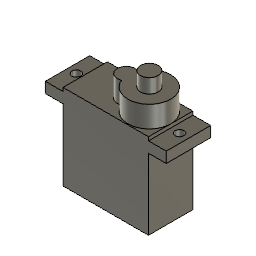
SG90 (Autodesk Fusion 360 design; units mm, degrees)
part number: 2026-08-23-17-35-19-332
Autodesk Fusion 360 part; units mm, degrees
note: some values were not read from the file. Set by a fixed rule: which sketch regions a step uses.
sketch "Sketch1" plane through (0, 0, 0) normal (0, 0, 1) x (1, 0, 0)
  line L0 (12, 6.25) -> (-12, 6.25)
  line L1 (-12, 6.25) -> (-12, -6.25)
  line L2 (-12, -6.25) -> (12, -6.25)
  line L3 (12, -6.25) -> (12, 6.25)
  line L4 (12, 6.25) -> (-12, -6.25) construction
  line L5 (-12, 6.25) -> (12, -6.25) construction
  line L6 (12, 6.25) -> (17, 6.25)
  line L7 (17, 6.25) -> (17, -6.25)
  line L8 (12, -6.25) -> (17, -6.25)
  line L9 (-12, 6.25) -> (-17, 6.25)
  line L10 (-17, 6.25) -> (-17, -6.25)
  line L11 (-17, -6.25) -> (-12, -6.25)
  dimension "d1" = 24
  dimension "d2" = 12.5
  dimension "d3" = 5
  dimension "d4" = 5
  constraint horizontal L0
  constraint perpendicular L0 L1
  constraint parallel L0 L2
  constraint parallel L1 L3
  constraint coincident L4 origin
  constraint coincident L5 origin
  constraint perpendicular L3 L6
  constraint perpendicular L2 L7
  constraint perpendicular L7 L8
  constraint perpendicular L1 L9
  constraint perpendicular L0 L10
  constraint perpendicular L1 L11
  measures "d1" distance of L1.end L2.end
  measures "d2" distance of L0.end L1.end
  measures "d3" distance of L0.start L6.end
  measures "d4" distance of L0.end L9.end
extrude "Extrude1" add sketch "Sketch1" along normal blind 24 contours L0 L1 L2 L3
sketch "Sketch2" plane through (0, -6.25, 0) normal (0, -1, 0) x (1, 0, 0)
  line L0 (-12, 0) -> (12, 0)
  line L1 (12, 0) -> (12, 24)
  line L2 (12, 24) -> (-12, 24)
  line L3 (-12, 24) -> (-12, 0)
  line L4 (12, 24) -> (12, 23)
  line L5 (12, 23) -> (17, 23)
  line L6 (17, 23) -> (17, 20)
  line L7 (17, 20) -> (12, 20)
  line L8 (-12, 24) -> (-12, 23)
  line L9 (-12, 23) -> (-17, 23)
  line L10 (-17, 23) -> (-17, 20)
  line L11 (-17, 20) -> (-12, 20)
  dimension "d7" = 1
  dimension "d8" = 5
  dimension "d9" = 3
  dimension "d10" = 1
  dimension "d11" = 5
  dimension "d12" = 3
  constraint coincident L1.end L2.start
  constraint perpendicular L2 L4
  constraint perpendicular L1 L5
  constraint perpendicular L5 L6
  constraint coincident L1 L7.end
  constraint perpendicular L1 L7
  constraint coincident L2.end L3.start
  constraint perpendicular L2 L8
  constraint perpendicular L3 L9
  constraint perpendicular L9 L10
  constraint coincident L3 L11.end
  constraint perpendicular L3 L11
  measures "d7" distance of L1.end L4.end
  measures "d8" distance of L4.end L5.end
  measures "d9" distance of L5.end L6.end
  measures "d10" distance of L2.end L8.end
  measures "d11" distance of L8.end L9.end
  measures "d12" distance of L9.end L10.end
extrude "Extrude2" add sketch "Sketch2" against normal up to surface (12.5 mm away) contours L3 L9 L10 L11 | L1 L5 L6 L7
sketch "Sketch3" plane through (0, 0, 24) normal (0, 0, 1) x (-1, 0, 0)
  line L0 (-12, 6.25) -> (-12, -6.25)
  line L1 (-12, -6.25) -> (12, -6.25)
  line L2 (12, -6.25) -> (12, 6.25)
  line L3 (12, 6.25) -> (-12, 6.25)
  circle A0 centre (-6, 0) radius 6
  circle A1 centre (0.5, 0) radius 2.5
  dimension "d15" = 12
  dimension "d16" = 5
  dimension "d17" = 6.5
  constraint tangent L0 A0
  measures "d15" diameter of A0
  measures "d16" diameter of A1
  measures "d17" distance of A0.centre A1.centre
extrude "Extrude3" add sketch "Sketch3" along normal blind 6 contours A0 A1 | A0 A1 | A0 A1
sketch "Sketch4" plane through (0, 0, 30) normal (0, 0, 1) x (-1, 0, 0)
  arc A0 (-0.4615, -2.3077) -> (-0.4615, 2.3077) centre (0.5, 0) ccw
  arc A1 (-0.4615, 2.3077) -> (-0.4615, -2.3077) centre (-6, 0) ccw
  circle A2 centre (-6, 0) radius 2.5
  dimension "d20" = 5
  constraint concentric A1 A2
  measures "d20" diameter of A2
extrude "Extrude4" add sketch "Sketch4" along normal blind 4 contours A2
sketch "Sketch5" plane through (0, 0, 23) normal (0, 0, 1) x (-1, 0, 0)
  line L0 (-17, -6.25) -> (-12, -6.25)
  line L1 (-12, -6.25) -> (-12, 6.25)
  line L2 (-12, 6.25) -> (-17, 6.25)
  line L3 (-17, 6.25) -> (-17, -6.25)
  circle A0 centre (-14.5, 0) radius 1.25
  dimension "d23" = 2.5
  dimension "d24" = 2.5
  measures "d23" diameter of A0
  measures "d24" distance of L3 A0.centre
sketch "Sketch6" plane through (0, 0, 23) normal (0, 0, 1) x (-1, 0, 0)
  line L0 (12, -6.25) -> (17, -6.25)
  line L1 (17, -6.25) -> (17, 6.25)
  line L2 (17, 6.25) -> (12, 6.25)
  line L3 (12, 6.25) -> (12, -6.25)
  circle A0 centre (14.5, 0) radius 1.25
  dimension "d25" = 2.5
  dimension "d26" = 2.5
  measures "d25" diameter of A0
  measures "d26" distance of L1 A0.centre
extrude "Extrude5" cut sketch "Sketch6" sketch "Sketch5" against normal blind 3 contours A0 of sketch 2 contours A0
